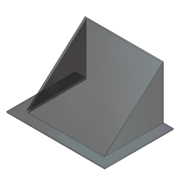
# Autodesk Inventor part: Panel_ShooterShroud
Saved by Autodesk Inventor 2012 (Build 160160000, 160)
## iProperties
Created: 2012-01-26
Part Number: Panel_ShooterShroud
Material: Polycarbonate, Smoke
Document SubType Name: Modeling
Designer: JesseK
Mass: 290.337 g
Surface Area: 1562.32 cm^2
Volume: 241.948 cm^3
Density: 1.2 g/cm^3
Author: JesseK
Autodesk Inventor part; units mm, degrees
ref_plane "YZ Plane" through (0, 0, 0) normal (1, 0, 0) x (0, 1, 0)
ref_plane "XZ Plane" through (0, 0, 0) normal (0, 1, 0) x (-1, 0, 0)
ref_plane "XY Plane" through (0, 0, 0) normal (0, 0, 1) x (1, 0, 0)
sketch "Sketch1" plane through (0, 0, 0) normal (0, 0, 1) x (1, 0, 0)
  line L0 (0, 0) -> (254, 0)
  line L1 (254, 0) -> (254, 139.7)
  line L2 (254, 139.7) -> (0, 139.7)
  line L3 (0, 139.7) -> (0, 0)
  dimension "d0" = 254
  dimension "d1" = 139.7
  constraints: 8 end point, 2 parallel, 1 horizontal, 1 perpendicular
  measures "d0" distance of L0.start L0.end
  measures "d1" distance of L2.end L0.start
extrude "Extrusion1" add sketch "Sketch1" along normal blind 177.8
sketch "Sketch4" plane through (254, 0, 0) normal (1, 0, 0) x (0, 0, -1)
  line L0 (-177.8, 139.7) -> (-177.8, 0) projected
  line L1 (0, 0) -> (-177.8, 0) projected
  line L2 (0, 139.7) -> (-177.8, 139.7)
  line L3 (-177.8, 139.7) -> (-177.8, 3.175)
  line L4 (-177.8, 3.175) -> (-152.4, 3.175)
  line L5 (-152.4, 3.175) -> (0, 139.7)
  dimension "d10" = 3.175
  dimension "d11" = 25.4
  constraints: 8 end point, 2 horizontal, 1 point on line
  measures "d10" distance between parallel lines of L1 L4
  measures "d11" distance of L3.end L4.end
extrude "Extrusion3" cut sketch "Sketch4" against normal through all
sketch "Sketch5" plane through (0, 0, 0) normal (0, 0, -1) x (-1, 0, 0)
  line L0 (0, 0) -> (-254, 0) projected
  line L1 (0, 139.7) -> (0, 0) projected
  line L2 (-254, 139.7) -> (-228.6, 139.7)
  line L3 (-228.6, 139.7) -> (-228.6, 3.175)
  line L4 (-228.6, 3.175) -> (-254, 3.175)
  line L5 (-254, 3.175) -> (-254, 139.7)
  line L6 (0, 139.7) -> (-25.4, 139.7)
  line L7 (-25.4, 139.7) -> (-25.4, 3.175)
  line L8 (-25.4, 3.175) -> (0, 3.175)
  line L9 (0, 3.175) -> (0, 139.7)
  dimension "d15" = 3.175
  dimension "d16" = 25.4
  constraints: 16 end point, 4 parallel, 2 collinear, 2 horizontal, 2 perpendicular
  measures "d15" distance between parallel lines of L0 L8
  measures "d16" distance between parallel lines of L1 L7
extrude "Extrusion4" cut sketch "Sketch5" against normal through all
shell "Shell1" thickness 3.175 removed faces 2 at (160.8667, 48.6833, 0) at (84.6667, 0, 59.2667)
body "Solid1"
